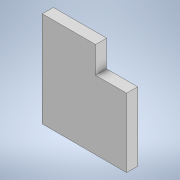
# Autodesk Inventor part: base box
Saved by Autodesk Inventor 2022 (Build 260153000, 153)
## iProperties
Created: 2022-07-18
Part Number: base box
Material: Generic
Document SubType Name: Modeling
Designer: yashm
Density: 1 g/cm^3
Appearance: Default
Author: yashm
Autodesk Inventor part; units mm, degrees
ref_plane "YZ Plane" through (0, 0, 0) normal (1, 0, 0) x (0, 1, 0)
ref_plane "XZ Plane" through (0, 0, 0) normal (0, 1, 0) x (-1, 0, 0)
ref_plane "XY Plane" through (0, 0, 0) normal (0, 0, 1) x (1, 0, 0)
sketch "Sketch1" plane through (0, 0, 0) normal (0, 0, 1) x (1, 0, 0)
  line L0 (0, 0) -> (0, 215)
  line L1 (0, 215) -> (120, 215)
  line L2 (120, 215) -> (120, 155)
  line L3 (120, 155) -> (190, 155)
  line L4 (190, 155) -> (190, 0)
  line L5 (190, 0) -> (0, 0)
  dimension "d1" = 155
  dimension "d2" = 60
  dimension "d3" = 120
  dimension "d4" = 70
  constraints: 12 end point, 5 perpendicular, 1 vertical
  measures "d1" distance of L3.end L4.end
  measures "d2" distance of L1.end L2.end
  measures "d3" distance of L0.end L1.end
  measures "d4" distance of L2.end L3.end
extrude "Extrusion1" add sketch "Sketch1" along normal blind 25
body "Solid1"
